# Autodesk Inventor part: straight
Saved by Autodesk Inventor 2021 (Build 250183000, 183)
## iProperties
Created: 2021-01-02
Part Number: straight
Material: Generic
Document SubType Name: Modeling
Designer: Tomasz
Density: 1 g/cm^3
Appearance: Default
Author: Tomasz
Autodesk Inventor part; units mm, degrees
ref_plane "YZ Plane" through (0, 0, 0) normal (1, 0, 0) x (0, 1, 0)
ref_plane "XZ Plane" through (0, 0, 0) normal (0, 1, 0) x (-1, 0, 0)
ref_plane "XY Plane" through (0, 0, 0) normal (0, 0, 1) x (1, 0, 0)
sketch "Sketch1" plane through (0, 0, 0) normal (0, 1, 0) x (-1, 0, 0)
  line L0 (275, 0) -> (-275, 0)
  line L1 (-275, 0) -> (-275, -720)
  line L2 (-275, -720) -> (275, -720)
  line L3 (275, -720) -> (275, 0)
  line L4 (255, 0) -> (255, -720)
  line L5 (-255, -720) -> (-255, 0)
  point P0 (0, 0)
  point P1 (0, 0)
  dimension "d0" = 550
  dimension "d1" = 720
  dimension "d4" = 20
  dimension "d5" = 20
  constraints: 12 end point, 4 point on line, 3 perpendicular, 2 parallel, 1 coincident, 1 horizontal, 1 midpoint
  measures "d0" distance of L2.end L1.end
  measures "d1" distance of L1.end L0.end
  measures "d4" distance between parallel lines of L1 L5
  measures "d5" distance between parallel lines of L3 L4
extrude "Extrusion1" add sketch "Sketch1" along normal blind 3
extrude "Extrusion2" add sketch "Sketch1" along normal blind 3.1 contours L3 L2 L4 L0 | L5 L2 L1 L0
equation "\"d0\" = track_width"
equation "\"d4\" = curb_width"
equation "\"d5\" = curb_width"
equation "\"d2\" = track_height"
equation "\"d6\" = track_height + curb_height"
equation "\"track_width\" = 550"
equation "\"curb_width\" = 20"
equation "\"track_height\" = 3"
equation "\"curb_height\" = 0.1"
body "Solid1"
